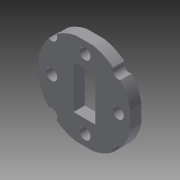
# Autodesk Inventor part: WG18FLANGECutDown
Saved by Autodesk Inventor 2015 (Build 190159000, 159)
## iProperties
Created: 2014-03-25
Part Number: WG18FLANGECutDown
Material: Generic
Document SubType Name: Modeling
Designer: jad211
Density: 1 g/cm^3
Appearance: Default
Author: jad211
Autodesk Inventor part; units mm, degrees
ref_plane "YZ Plane" through (0, 0, 0) normal (1, 0, 0) x (0, 1, 0)
ref_plane "XZ Plane" through (0, 0, 0) normal (0, 1, 0) x (-1, 0, 0)
ref_plane "XY Plane" through (0, 0, 0) normal (0, 0, 1) x (1, 0, 0)
sketch "Sketch3" plane through (0, 0, 0) normal (0, 0, 1) x (1, 0, 0)
  line L0 (-15.7, -16.7) -> (15.7, -16.7)
  line L1 (16.7, -15.7) -> (16.7, 15.7)
  line L2 (15.7, 16.7) -> (-15.7, 16.7)
  line L3 (-16.7, 15.7) -> (-16.7, -15.7)
  line L4 (-15.7, 16.7) -> (-16.7, 15.7)
  line L5 (15.7, 16.7) -> (16.7, 15.7)
  line L6 (16.7, -15.7) -> (15.7, -16.7)
  line L7 (-16.7, -15.7) -> (-15.7, -16.7)
  line L8 (-3.9497, -7.8994) -> (3.9497, -7.8994)
  line L9 (3.9497, -7.8994) -> (3.9497, 7.8994)
  line L10 (3.9497, 7.8994) -> (-3.9497, 7.8994)
  line L11 (-3.9497, 7.8994) -> (-3.9497, -7.8994)
  circle A0 centre (-11.9482, 12.625) radius 2.045
  circle A1 centre (12.3318, 12.625) radius 2.045
  line L12 (0, -16.7) -> (0, 16.7) construction
  circle A2 centre (-11.9482, -12.625) radius 2.045
  circle A3 centre (12.3318, -12.625) radius 2.045
  line L13 (12.3318, 12.625) -> (-11.9482, 12.625) construction
  line L14 (-11.9482, 12.625) -> (-11.9482, -12.625) construction
  line L15 (-11.9482, -12.625) -> (12.3318, -12.625) construction
  line L16 (12.3318, -12.625) -> (12.3318, 12.625) construction
  line L17 (-16.7, 0) -> (16.7, 0) construction
  circle A4 centre (0, 0) radius 18.4 construction
  circle A5 centre (-11.9482, 0) radius 2.045
  circle A6 centre (0.1918, 12.625) radius 2.045
  circle A7 centre (12.3318, 0) radius 2.045
  circle A8 centre (0.1918, -12.625) radius 2.045
  dimension "d10" = 7.8994
  dimension "d11" = 15.7988
  dimension "d12" = 4.09
  dimension "d13" = 4.09
  dimension "d17" = 4.09
  dimension "d19" = 24.28
  dimension "d20" = 25.25
  dimension "d21" = 4.09
  dimension "d22" = 12.625
  dimension "d26" = 36.8
  dimension "d27" = 4.09
  dimension "d28" = 4.09
  dimension "d29" = 4.09
  dimension "d33" = 4.09
  constraints: 37 end point, 9 centre point, 8 midpoint, 6 perpendicular, 4 parallel, 2 horizontal, 2 point on line
  measures "d10" distance of L10.end L9.end
  measures "d11" distance of L9.end L8.end
  measures "d12" diameter of A0
  measures "d13" diameter of A1
  measures "d17" diameter of A2
  measures "d19" distance of L13.start L13.end
  measures "d20" distance of L14.end L13.end
  measures "d21" diameter of A3
  measures "d22" distance from line of L17.start L13
  measures "d26" diameter of A4
  measures "d27" diameter of A5
  measures "d28" diameter of A6
  measures "d29" diameter of A7
  measures "d33" diameter of A8
sketch "Sketch4" plane through (0, 0, 0) normal (0, 0, 1) x (1, 0, 0)
  circle A0 centre (0, 0) radius 17
  dimension "d32" = 34
  constraints: 1 centre point, 1 coincident
  measures "d32" diameter of A0
extrude "Extrusion3" add sketch "Sketch3" along normal blind 4.1
extrude "Extrusion4" cut sketch "Sketch4" along normal blind 4.1 keep common part
body "Solid3"
